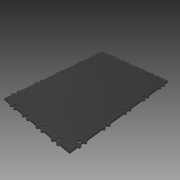
# Autodesk Inventor part: bottom
Saved by Autodesk Inventor 2014 (Build 180170000, 170)
## iProperties
Created: 2013-12-07
Part Number: bottom
Material: Generic
Document SubType Name: Modeling
Designer: buben
Density: 1 g/cm^3
Appearance: Anodized - Dark Gray
Author: buben
Subject: Laser Cutted
Autodesk Inventor part; units mm, degrees
ref_plane "YZ Plane" through (0, 0, 0) normal (1, 0, 0) x (0, 1, 0)
ref_plane "XZ Plane" through (0, 0, 0) normal (0, 1, 0) x (-1, 0, 0)
ref_plane "XY Plane" through (0, 0, 0) normal (0, 0, 1) x (1, 0, 0)
sketch "Sketch1" plane through (0, 0, 0) normal (0, 0, 1) x (1, 0, 0)
  line L0 (0, 0) -> (335, 0)
  line L1 (335, 0) -> (335, 489)
  line L2 (335, 489) -> (0, 489)
  line L3 (0, 489) -> (0, 0)
  dimension "d0" = 335
  dimension "d1" = 489
  constraints: 8 end point, 2 parallel, 1 horizontal, 1 perpendicular
  measures "d0" distance of L0.start L0.end
  measures "d1" distance of L2.end L0.start
extrude "Extrusion1" add sketch "Sketch1" along normal blind 6
sketch "Sketch6" plane through (0, 0, 6) normal (0, 0, 1) x (1, 0, 0)
  line L0 (0, 0) -> (335, 0) projected
  line L1 (335, 0) -> (335, 489) projected
  line L2 (335, 489) -> (0, 489) projected
  line L3 (0, 489) -> (0, 0) projected
  line L4 (55.45, 0) -> (59.95, 0)
  line L5 (59.95, 16.3) -> (55.45, 16.3)
  line L6 (62.45, 12.3) -> (62.45, 5)
  line L7 (52.95, 5) -> (52.95, 12.3)
  line L8 (55.45, 16.3) -> (55.45, 12.3)
  line L9 (55.45, 5) -> (55.45, 0)
  line L10 (59.95, 0) -> (59.95, 5)
  line L11 (59.95, 12.3) -> (59.95, 16.3)
  line L12 (62.45, 5) -> (59.95, 5)
  line L13 (55.45, 5) -> (52.95, 5)
  line L14 (52.95, 12.3) -> (55.45, 12.3)
  line L15 (59.95, 12.3) -> (62.45, 12.3)
  line L16 (128.65, 0) -> (133.15, 0)
  line L17 (133.15, 16.3) -> (128.65, 16.3)
  line L18 (135.65, 12.3) -> (135.65, 5)
  line L19 (126.15, 5) -> (126.15, 12.3)
  line L20 (128.65, 16.3) -> (128.65, 12.3)
  line L21 (128.65, 5) -> (128.65, 0)
  line L22 (133.15, 0) -> (133.15, 5)
  line L23 (133.15, 12.3) -> (133.15, 16.3)
  line L24 (135.65, 5) -> (133.15, 5)
  line L25 (128.65, 5) -> (126.15, 5)
  line L26 (126.15, 12.3) -> (128.65, 12.3)
  line L27 (133.15, 12.3) -> (135.65, 12.3)
  line L28 (201.85, 0) -> (206.35, 0)
  line L29 (206.35, 16.3) -> (201.85, 16.3)
  line L30 (208.85, 12.3) -> (208.85, 5)
  line L31 (199.35, 5) -> (199.35, 12.3)
  line L32 (201.85, 16.3) -> (201.85, 12.3)
  line L33 (201.85, 5) -> (201.85, 0)
  line L34 (206.35, 0) -> (206.35, 5)
  line L35 (206.35, 12.3) -> (206.35, 16.3)
  line L36 (208.85, 5) -> (206.35, 5)
  line L37 (201.85, 5) -> (199.35, 5)
  line L38 (199.35, 12.3) -> (201.85, 12.3)
  line L39 (206.35, 12.3) -> (208.85, 12.3)
  line L40 (275.05, 0) -> (279.55, 0)
  line L41 (279.55, 16.3) -> (275.05, 16.3)
  line L42 (282.05, 12.3) -> (282.05, 5)
  line L43 (272.55, 5) -> (272.55, 12.3)
  line L44 (275.05, 16.3) -> (275.05, 12.3)
  line L45 (275.05, 5) -> (275.05, 0)
  line L46 (279.55, 0) -> (279.55, 5)
  line L47 (279.55, 12.3) -> (279.55, 16.3)
  line L48 (282.05, 5) -> (279.55, 5)
  line L49 (275.05, 5) -> (272.55, 5)
  line L50 (272.55, 12.3) -> (275.05, 12.3)
  line L51 (279.55, 12.3) -> (282.05, 12.3)
  line L52 (0, 244.5) -> (335, 244.5) construction
  line L53 (55.45, 489) -> (59.95, 489)
  line L54 (59.95, 472.7) -> (55.45, 472.7)
  line L55 (62.45, 476.7) -> (62.45, 484)
  line L56 (52.95, 484) -> (52.95, 476.7)
  line L57 (55.45, 472.7) -> (55.45, 476.7)
  line L58 (55.45, 484) -> (55.45, 489)
  line L59 (59.95, 489) -> (59.95, 484)
  line L60 (59.95, 476.7) -> (59.95, 472.7)
  line L61 (62.45, 484) -> (59.95, 484)
  line L62 (55.45, 484) -> (52.95, 484)
  line L63 (52.95, 476.7) -> (55.45, 476.7)
  line L64 (59.95, 476.7) -> (62.45, 476.7)
  line L65 (128.65, 484) -> (126.15, 484)
  line L66 (135.65, 484) -> (133.15, 484)
  line L67 (128.65, 484) -> (128.65, 489)
  line L68 (128.65, 489) -> (133.15, 489)
  line L69 (133.15, 489) -> (133.15, 484)
  line L70 (126.15, 476.7) -> (128.65, 476.7)
  line L71 (126.15, 484) -> (126.15, 476.7)
  line L72 (133.15, 476.7) -> (135.65, 476.7)
  line L73 (135.65, 476.7) -> (135.65, 484)
  line L74 (128.65, 472.7) -> (128.65, 476.7)
  line L75 (133.15, 476.7) -> (133.15, 472.7)
  line L76 (133.15, 472.7) -> (128.65, 472.7)
  line L77 (201.85, 484) -> (199.35, 484)
  line L78 (208.85, 484) -> (206.35, 484)
  line L79 (201.85, 484) -> (201.85, 489)
  line L80 (201.85, 489) -> (206.35, 489)
  line L81 (206.35, 489) -> (206.35, 484)
  line L82 (199.35, 476.7) -> (201.85, 476.7)
  line L83 (199.35, 484) -> (199.35, 476.7)
  line L84 (206.35, 476.7) -> (208.85, 476.7)
  line L85 (208.85, 476.7) -> (208.85, 484)
  line L86 (201.85, 472.7) -> (201.85, 476.7)
  line L87 (206.35, 476.7) -> (206.35, 472.7)
  line L88 (206.35, 472.7) -> (201.85, 472.7)
  line L89 (275.05, 484) -> (272.55, 484)
  line L90 (282.05, 484) -> (279.55, 484)
  line L91 (275.05, 484) -> (275.05, 489)
  line L92 (275.05, 489) -> (279.55, 489)
  line L93 (279.55, 489) -> (279.55, 484)
  line L94 (272.55, 476.7) -> (275.05, 476.7)
  line L95 (272.55, 484) -> (272.55, 476.7)
  line L96 (279.55, 476.7) -> (282.05, 476.7)
  line L97 (282.05, 476.7) -> (282.05, 484)
  line L98 (275.05, 472.7) -> (275.05, 476.7)
  line L99 (279.55, 476.7) -> (279.55, 472.7)
  line L100 (279.55, 472.7) -> (275.05, 472.7)
  line L101 (16.3, 47.75) -> (16.3, 43.25)
  line L102 (0, 43.25) -> (0, 47.75)
  line L103 (5, 50.25) -> (12.3, 50.25)
  line L104 (12.3, 40.75) -> (5, 40.75)
  line L105 (5, 40.75) -> (5, 43.25)
  line L106 (5, 47.75) -> (5, 50.25)
  line L107 (12.3, 50.25) -> (12.3, 47.75)
  line L108 (12.3, 43.25) -> (12.3, 40.75)
  line L109 (0, 47.75) -> (5, 47.75)
  line L110 (12.3, 47.75) -> (16.3, 47.75)
  line L111 (16.3, 43.25) -> (12.3, 43.25)
  line L112 (5, 43.25) -> (0, 43.25)
  line L113 (167.5, 489) -> (167.5, 0) construction
  line L114 (16.3, 147.25) -> (16.3, 142.75)
  line L115 (0, 142.75) -> (0, 147.25)
  line L116 (5, 149.75) -> (12.3, 149.75)
  line L117 (12.3, 140.25) -> (5, 140.25)
  line L118 (5, 140.25) -> (5, 142.75)
  line L119 (5, 147.25) -> (5, 149.75)
  line L120 (12.3, 149.75) -> (12.3, 147.25)
  line L121 (12.3, 142.75) -> (12.3, 140.25)
  line L122 (0, 147.25) -> (5, 147.25)
  line L123 (12.3, 147.25) -> (16.3, 147.25)
  line L124 (16.3, 142.75) -> (12.3, 142.75)
  line L125 (5, 142.75) -> (0, 142.75)
  line L126 (16.3, 246.75) -> (16.3, 242.25)
  line L127 (0, 242.25) -> (0, 246.75)
  line L128 (5, 249.25) -> (12.3, 249.25)
  line L129 (12.3, 239.75) -> (5, 239.75)
  line L130 (5, 239.75) -> (5, 242.25)
  line L131 (5, 246.75) -> (5, 249.25)
  line L132 (12.3, 249.25) -> (12.3, 246.75)
  line L133 (12.3, 242.25) -> (12.3, 239.75)
  line L134 (0, 246.75) -> (5, 246.75)
  line L135 (12.3, 246.75) -> (16.3, 246.75)
  line L136 (16.3, 242.25) -> (12.3, 242.25)
  line L137 (5, 242.25) -> (0, 242.25)
  line L138 (16.3, 346.25) -> (16.3, 341.75)
  line L139 (0, 341.75) -> (0, 346.25)
  line L140 (5, 348.75) -> (12.3, 348.75)
  line L141 (12.3, 339.25) -> (5, 339.25)
  line L142 (5, 339.25) -> (5, 341.75)
  line L143 (5, 346.25) -> (5, 348.75)
  line L144 (12.3, 348.75) -> (12.3, 346.25)
  line L145 (12.3, 341.75) -> (12.3, 339.25)
  line L146 (0, 346.25) -> (5, 346.25)
  line L147 (12.3, 346.25) -> (16.3, 346.25)
  line L148 (16.3, 341.75) -> (12.3, 341.75)
  line L149 (5, 341.75) -> (0, 341.75)
  line L150 (16.3, 445.75) -> (16.3, 441.25)
  line L151 (0, 441.25) -> (0, 445.75)
  line L152 (5, 448.25) -> (12.3, 448.25)
  line L153 (12.3, 438.75) -> (5, 438.75)
  line L154 (5, 438.75) -> (5, 441.25)
  line L155 (5, 445.75) -> (5, 448.25)
  line L156 (12.3, 448.25) -> (12.3, 445.75)
  line L157 (12.3, 441.25) -> (12.3, 438.75)
  line L158 (0, 445.75) -> (5, 445.75)
  line L159 (12.3, 445.75) -> (16.3, 445.75)
  line L160 (16.3, 441.25) -> (12.3, 441.25)
  line L161 (5, 441.25) -> (0, 441.25)
  line L162 (318.7, 47.75) -> (318.7, 43.25)
  line L163 (335, 43.25) -> (335, 47.75)
  line L164 (330, 50.25) -> (322.7, 50.25)
  line L165 (322.7, 40.75) -> (330, 40.75)
  line L166 (330, 40.75) -> (330, 43.25)
  line L167 (330, 47.75) -> (330, 50.25)
  line L168 (322.7, 50.25) -> (322.7, 47.75)
  line L169 (322.7, 43.25) -> (322.7, 40.75)
  line L170 (335, 47.75) -> (330, 47.75)
  line L171 (322.7, 47.75) -> (318.7, 47.75)
  line L172 (318.7, 43.25) -> (322.7, 43.25)
  line L173 (330, 43.25) -> (335, 43.25)
  line L174 (322.7, 147.25) -> (318.7, 147.25)
  line L175 (318.7, 147.25) -> (318.7, 142.75)
  line L176 (318.7, 142.75) -> (322.7, 142.75)
  line L177 (322.7, 149.75) -> (322.7, 147.25)
  line L178 (322.7, 142.75) -> (322.7, 140.25)
  line L179 (322.7, 140.25) -> (330, 140.25)
  line L180 (330, 149.75) -> (322.7, 149.75)
  line L181 (330, 140.25) -> (330, 142.75)
  line L182 (330, 147.25) -> (330, 149.75)
  line L183 (335, 147.25) -> (330, 147.25)
  line L184 (335, 142.75) -> (335, 147.25)
  line L185 (330, 142.75) -> (335, 142.75)
  line L186 (322.7, 246.75) -> (318.7, 246.75)
  line L187 (318.7, 246.75) -> (318.7, 242.25)
  line L188 (318.7, 242.25) -> (322.7, 242.25)
  line L189 (322.7, 249.25) -> (322.7, 246.75)
  line L190 (322.7, 242.25) -> (322.7, 239.75)
  line L191 (322.7, 239.75) -> (330, 239.75)
  line L192 (330, 249.25) -> (322.7, 249.25)
  line L193 (330, 239.75) -> (330, 242.25)
  line L194 (330, 246.75) -> (330, 249.25)
  line L195 (335, 246.75) -> (330, 246.75)
  line L196 (335, 242.25) -> (335, 246.75)
  line L197 (330, 242.25) -> (335, 242.25)
  line L198 (322.7, 346.25) -> (318.7, 346.25)
  line L199 (318.7, 346.25) -> (318.7, 341.75)
  line L200 (318.7, 341.75) -> (322.7, 341.75)
  line L201 (322.7, 348.75) -> (322.7, 346.25)
  line L202 (322.7, 341.75) -> (322.7, 339.25)
  line L203 (322.7, 339.25) -> (330, 339.25)
  line L204 (330, 348.75) -> (322.7, 348.75)
  line L205 (330, 339.25) -> (330, 341.75)
  line L206 (330, 346.25) -> (330, 348.75)
  line L207 (335, 346.25) -> (330, 346.25)
  line L208 (335, 341.75) -> (335, 346.25)
  line L209 (330, 341.75) -> (335, 341.75)
  line L210 (322.7, 445.75) -> (318.7, 445.75)
  line L211 (318.7, 445.75) -> (318.7, 441.25)
  line L212 (318.7, 441.25) -> (322.7, 441.25)
  line L213 (322.7, 448.25) -> (322.7, 445.75)
  line L214 (322.7, 441.25) -> (322.7, 438.75)
  line L215 (322.7, 438.75) -> (330, 438.75)
  line L216 (330, 448.25) -> (322.7, 448.25)
  line L217 (330, 438.75) -> (330, 441.25)
  line L218 (330, 445.75) -> (330, 448.25)
  line L219 (335, 445.75) -> (330, 445.75)
  line L220 (335, 441.25) -> (335, 445.75)
  line L221 (330, 441.25) -> (335, 441.25)
  point P0 (57.7, 16.3)
  point P1 (130.9, 16.3)
  point P2 (204.1, 16.3)
  point P3 (277.3, 16.3)
  point P4 (57.7, 472.7)
  point P5 (130.9, 472.7)
  point P6 (204.1, 472.7)
  point P7 (277.3, 472.7)
  point P8 (16.3, 45.5)
  point P9 (16.3, 145)
  point P10 (16.3, 244.5)
  point P11 (16.3, 344)
  point P12 (16.3, 443.5)
  point P13 (318.7, 45.5)
  point P14 (318.7, 145)
  point P15 (318.7, 244.5)
  point P16 (318.7, 344)
  point P17 (318.7, 443.5)
  dimension "d66" = 4.5
  dimension "d67" = 7.3
  dimension "d68" = 5
  dimension "d69" = 4
  dimension "d70" = 2.5
  dimension "d71" = 2.5
  dimension "d72" = 57.7
  dimension "d75" = 73.2
  dimension "d80" = 4.5
  dimension "d81" = 7.3
  dimension "d82" = 5
  dimension "d83" = 4
  dimension "d84" = 2.5
  dimension "d85" = 2.5
  dimension "d86" = 45.5
  dimension "d89" = 99.5
  constraints: 436 end point, 117 symmetric about line, 20 parallel, 9 collinear, 8 perpendicular, 7 horizontal, 6 midpoint, 1 point on line, 1 vertical, 175 other
  measures "d66" distance of L5.start L5.end
  measures "d67" distance of L6.start L6.end
  measures "d68" distance of L4.end L10.end
  measures "d69" distance of L11.start L5.start
  measures "d70" distance of L7.end L8.end
  measures "d71" distance of L11.start L6.start
  measures "d72" distance from line of L3 point (57.7, 16.3)
  measures "d75" distance of L7.start L25.end
  measures "d80" distance of L101.start L101.end
  measures "d81" distance of L104.start L104.end
  measures "d82" distance of L105.end L102.start
  measures "d83" distance of L101.end L108.start
  measures "d84" distance of L104.end L105.end
  measures "d85" distance of L106.start L103.start
  measures "d86" distance from line of L0 point (16.3, 45.5)
  measures "d89" distance of L101.start L123.end
extrude "Extrusion6" cut sketch "Sketch6" against normal blind 6 contours L9 L13 L7 L14 L8 L5 L11 L15 L6 L12 L10 L0 | L3 L109 L106 L103 L107 L110 L101 L111 L108 L104 L105 L112 | L21 L25 L19 L26 L20 L17 L23 L27 L18 L24 L22 L0 | L3 L122 L119 L116 L120 L123 L114 L124 L121 L117 L118 L125 | L33 L37 L31 L38 L32 L29 L35 L39 L30 L36 L34 L0 | L3 L134 L131 L128 L132 L135 L126 L136 L133 L129 L130 L137 | L45 L49 L43 L50 L44 L41 L47 L51 L42 L48 L46 L0 | L3 L146 L143 L140 L144 L147 L138 L148 L145 L141 L142 L149 | L3 L158 L155 L152 L156 L159 L150 L160 L157 L153 L154 L161 | L173 L166 L165 L169 L172 L162 L171 L168 L164 L167 L170 L1 | L185 L181 L179 L178 L176 L175 L174 L177 L180 L182 L183 L1 | L2 L59 L61 L55 L64 L60 L54 L57 L63 L56 L62 L58 | L197 L193 L191 L190 L188 L187 L186 L189 L192 L194 L195 L1 | L2 L69 L66 L73 L72 L75 L76 L74 L70 L71 L65 L67 | L209 L205 L203 L202 L200 L199 L198 L201 L204 L206 L207 L1 | L2 L81 L78 L85 L84 L87 L88 L86 L82 L83 L77 L79 | L221 L217 L215 L214 L212 L211 L210 L213 L216 L218 L219 L1 | L2 L93 L90 L97 L96 L99 L100 L98 L94 L95 L89 L91
sketch "Sketch7" plane through (0, 0, 6) normal (0, 0, 1) x (1, 0, 0)
  line L0 (318.7, 242.25) -> (318.7, 246.75) projected
  line L1 (201.85, 489) -> (133.15, 489) projected
  line L2 (16.3, 246.75) -> (16.3, 242.25) projected
  line L3 (0, 142.75) -> (0, 47.75) projected
  line L4 (16.3, 47.75) -> (16.3, 43.25) projected
  line L5 (0, 43.25) -> (0, 0) projected
  line L6 (0, 0) -> (55.45, 0) projected
  line L7 (55.45, 16.3) -> (59.95, 16.3) projected
  line L8 (59.95, 0) -> (128.65, 0) projected
  line L9 (133.15, 0) -> (201.85, 0) projected
  line L10 (42.2, 0) -> (50.2, 0)
  line L11 (50.2, 0) -> (50.2, -4)
  line L12 (48.2, -6) -> (44.2, -6)
  line L13 (42.2, -4) -> (42.2, 0)
  line L14 (65.2, 0) -> (73.2, 0)
  line L15 (73.2, 0) -> (73.2, -4)
  line L16 (71.2, -6) -> (67.2, -6)
  line L17 (65.2, -4) -> (65.2, 0)
  line L18 (0, 38) -> (-4, 38)
  line L19 (-6, 36) -> (-6, 32)
  line L20 (-4, 30) -> (0, 30)
  line L21 (0, 30) -> (0, 38)
  line L22 (0, 61) -> (-4, 61)
  line L23 (-6, 59) -> (-6, 55)
  line L24 (-4, 53) -> (0, 53)
  line L25 (0, 53) -> (0, 61)
  arc A0 (-6, 55) -> (-4, 53) centre (-4, 55) ccw
  arc A1 (-4, 61) -> (-6, 59) centre (-4, 59) ccw
  arc A2 (-4, 38) -> (-6, 36) centre (-4, 36) ccw
  arc A3 (-6, 32) -> (-4, 30) centre (-4, 32) ccw
  arc A4 (42.2, -4) -> (44.2, -6) centre (44.2, -4) ccw
  arc A5 (48.2, -6) -> (50.2, -4) centre (48.2, -4) ccw
  arc A6 (65.2, -4) -> (67.2, -6) centre (67.2, -4) ccw
  arc A7 (71.2, -6) -> (73.2, -4) centre (71.2, -4) ccw
  line L26 (167.5, 489) -> (167.5, 0) construction
  line L27 (115.4, 0) -> (123.4, 0)
  line L28 (123.4, 0) -> (123.4, -4)
  line L29 (121.4, -6) -> (117.4, -6)
  line L30 (115.4, -4) -> (115.4, 0)
  line L31 (138.4, 0) -> (146.4, 0)
  line L32 (146.4, 0) -> (146.4, -4)
  line L33 (144.4, -6) -> (140.4, -6)
  line L34 (138.4, -4) -> (138.4, 0)
  arc A8 (115.4, -4) -> (117.4, -6) centre (117.4, -4) ccw
  arc A9 (121.4, -6) -> (123.4, -4) centre (121.4, -4) ccw
  arc A10 (138.4, -4) -> (140.4, -6) centre (140.4, -4) ccw
  arc A11 (144.4, -6) -> (146.4, -4) centre (144.4, -4) ccw
  line L35 (188.6, 0) -> (196.6, 0)
  line L36 (196.6, 0) -> (196.6, -4)
  line L37 (194.6, -6) -> (190.6, -6)
  line L38 (188.6, -4) -> (188.6, 0)
  line L39 (211.6, 0) -> (219.6, 0)
  line L40 (219.6, 0) -> (219.6, -4)
  line L41 (217.6, -6) -> (213.6, -6)
  line L42 (211.6, -4) -> (211.6, 0)
  arc A12 (188.6, -4) -> (190.6, -6) centre (190.6, -4) ccw
  arc A13 (194.6, -6) -> (196.6, -4) centre (194.6, -4) ccw
  arc A14 (211.6, -4) -> (213.6, -6) centre (213.6, -4) ccw
  arc A15 (217.6, -6) -> (219.6, -4) centre (217.6, -4) ccw
  line L43 (261.8, 0) -> (269.8, 0)
  line L44 (269.8, 0) -> (269.8, -4)
  line L45 (267.8, -6) -> (263.8, -6)
  line L46 (261.8, -4) -> (261.8, 0)
  line L47 (284.8, 0) -> (292.8, 0)
  line L48 (292.8, 0) -> (292.8, -4)
  line L49 (290.8, -6) -> (286.8, -6)
  line L50 (284.8, -4) -> (284.8, 0)
  arc A16 (261.8, -4) -> (263.8, -6) centre (263.8, -4) ccw
  arc A17 (267.8, -6) -> (269.8, -4) centre (267.8, -4) ccw
  arc A18 (284.8, -4) -> (286.8, -6) centre (286.8, -4) ccw
  arc A19 (290.8, -6) -> (292.8, -4) centre (290.8, -4) ccw
  line L51 (0, 137.5) -> (-4, 137.5)
  line L52 (-6, 135.5) -> (-6, 131.5)
  line L53 (-4, 129.5) -> (0, 129.5)
  line L54 (0, 129.5) -> (0, 137.5)
  line L55 (0, 160.5) -> (-4, 160.5)
  line L56 (-6, 158.5) -> (-6, 154.5)
  line L57 (-4, 152.5) -> (0, 152.5)
  line L58 (0, 152.5) -> (0, 160.5)
  arc A20 (-6, 154.5) -> (-4, 152.5) centre (-4, 154.5) ccw
  arc A21 (-4, 160.5) -> (-6, 158.5) centre (-4, 158.5) ccw
  arc A22 (-4, 137.5) -> (-6, 135.5) centre (-4, 135.5) ccw
  arc A23 (-6, 131.5) -> (-4, 129.5) centre (-4, 131.5) ccw
  line L59 (0, 237) -> (-4, 237)
  line L60 (-6, 235) -> (-6, 231)
  line L61 (-4, 229) -> (0, 229)
  line L62 (0, 229) -> (0, 237)
  line L63 (0, 260) -> (-4, 260)
  line L64 (-6, 258) -> (-6, 254)
  line L65 (-4, 252) -> (0, 252)
  line L66 (0, 252) -> (0, 260)
  arc A24 (-6, 254) -> (-4, 252) centre (-4, 254) ccw
  arc A25 (-4, 260) -> (-6, 258) centre (-4, 258) ccw
  arc A26 (-4, 237) -> (-6, 235) centre (-4, 235) ccw
  arc A27 (-6, 231) -> (-4, 229) centre (-4, 231) ccw
  line L67 (0, 336.5) -> (-4, 336.5)
  line L68 (-6, 334.5) -> (-6, 330.5)
  line L69 (-4, 328.5) -> (0, 328.5)
  line L70 (0, 328.5) -> (0, 336.5)
  line L71 (0, 359.5) -> (-4, 359.5)
  line L72 (-6, 357.5) -> (-6, 353.5)
  line L73 (-4, 351.5) -> (0, 351.5)
  line L74 (0, 351.5) -> (0, 359.5)
  arc A28 (-6, 353.5) -> (-4, 351.5) centre (-4, 353.5) ccw
  arc A29 (-4, 359.5) -> (-6, 357.5) centre (-4, 357.5) ccw
  arc A30 (-4, 336.5) -> (-6, 334.5) centre (-4, 334.5) ccw
  arc A31 (-6, 330.5) -> (-4, 328.5) centre (-4, 330.5) ccw
  line L75 (0, 436) -> (-4, 436)
  line L76 (-6, 434) -> (-6, 430)
  line L77 (-4, 428) -> (0, 428)
  line L78 (0, 428) -> (0, 436)
  line L79 (0, 459) -> (-4, 459)
  line L80 (-6, 457) -> (-6, 453)
  line L81 (-4, 451) -> (0, 451)
  line L82 (0, 451) -> (0, 459)
  arc A32 (-6, 453) -> (-4, 451) centre (-4, 453) ccw
  arc A33 (-4, 459) -> (-6, 457) centre (-4, 457) ccw
  arc A34 (-4, 436) -> (-6, 434) centre (-4, 434) ccw
  arc A35 (-6, 430) -> (-4, 428) centre (-4, 430) ccw
  line L83 (335, 38) -> (339, 38)
  line L84 (341, 36) -> (341, 32)
  line L85 (339, 30) -> (335, 30)
  line L86 (335, 30) -> (335, 38)
  line L87 (335, 61) -> (339, 61)
  line L88 (341, 59) -> (341, 55)
  line L89 (339, 53) -> (335, 53)
  line L90 (335, 53) -> (335, 61)
  arc A36 (339, 53) -> (341, 55) centre (339, 55) ccw
  arc A37 (341, 59) -> (339, 61) centre (339, 59) ccw
  arc A38 (341, 36) -> (339, 38) centre (339, 36) ccw
  arc A39 (339, 30) -> (341, 32) centre (339, 32) ccw
  line L91 (339, 152.5) -> (335, 152.5)
  line L92 (335, 160.5) -> (339, 160.5)
  line L93 (335, 152.5) -> (335, 160.5)
  arc A40 (341, 158.5) -> (339, 160.5) centre (339, 158.5) ccw
  line L94 (341, 158.5) -> (341, 154.5)
  arc A41 (339, 152.5) -> (341, 154.5) centre (339, 154.5) ccw
  arc A42 (341, 135.5) -> (339, 137.5) centre (339, 135.5) ccw
  line L95 (341, 135.5) -> (341, 131.5)
  arc A43 (339, 129.5) -> (341, 131.5) centre (339, 131.5) ccw
  line L96 (335, 137.5) -> (339, 137.5)
  line L97 (339, 129.5) -> (335, 129.5)
  line L98 (335, 129.5) -> (335, 137.5)
  line L99 (339, 252) -> (335, 252)
  line L100 (335, 260) -> (339, 260)
  line L101 (335, 252) -> (335, 260)
  arc A44 (341, 258) -> (339, 260) centre (339, 258) ccw
  line L102 (341, 258) -> (341, 254)
  arc A45 (339, 252) -> (341, 254) centre (339, 254) ccw
  arc A46 (341, 235) -> (339, 237) centre (339, 235) ccw
  line L103 (341, 235) -> (341, 231)
  arc A47 (339, 229) -> (341, 231) centre (339, 231) ccw
  line L104 (335, 237) -> (339, 237)
  line L105 (339, 229) -> (335, 229)
  line L106 (335, 229) -> (335, 237)
  line L107 (339, 351.5) -> (335, 351.5)
  line L108 (335, 359.5) -> (339, 359.5)
  line L109 (335, 351.5) -> (335, 359.5)
  arc A48 (341, 357.5) -> (339, 359.5) centre (339, 357.5) ccw
  line L110 (341, 357.5) -> (341, 353.5)
  arc A49 (339, 351.5) -> (341, 353.5) centre (339, 353.5) ccw
  arc A50 (341, 334.5) -> (339, 336.5) centre (339, 334.5) ccw
  line L111 (341, 334.5) -> (341, 330.5)
  arc A51 (339, 328.5) -> (341, 330.5) centre (339, 330.5) ccw
  line L112 (335, 336.5) -> (339, 336.5)
  line L113 (339, 328.5) -> (335, 328.5)
  line L114 (335, 328.5) -> (335, 336.5)
  line L115 (339, 451) -> (335, 451)
  line L116 (335, 459) -> (339, 459)
  line L117 (335, 451) -> (335, 459)
  arc A52 (341, 457) -> (339, 459) centre (339, 457) ccw
  line L118 (341, 457) -> (341, 453)
  arc A53 (339, 451) -> (341, 453) centre (339, 453) ccw
  arc A54 (341, 434) -> (339, 436) centre (339, 434) ccw
  line L119 (341, 434) -> (341, 430)
  arc A55 (339, 428) -> (341, 430) centre (339, 430) ccw
  line L120 (335, 436) -> (339, 436)
  line L121 (339, 428) -> (335, 428)
  line L122 (335, 428) -> (335, 436)
  line L123 (16.3, 244.5) -> (318.7, 244.5) construction
  line L124 (42.2, 489) -> (50.2, 489)
  line L125 (50.2, 489) -> (50.2, 493)
  line L126 (48.2, 495) -> (44.2, 495)
  line L127 (42.2, 493) -> (42.2, 489)
  line L128 (65.2, 489) -> (73.2, 489)
  line L129 (73.2, 489) -> (73.2, 493)
  line L130 (71.2, 495) -> (67.2, 495)
  line L131 (65.2, 493) -> (65.2, 489)
  arc A56 (44.2, 495) -> (42.2, 493) centre (44.2, 493) ccw
  arc A57 (50.2, 493) -> (48.2, 495) centre (48.2, 493) ccw
  arc A58 (67.2, 495) -> (65.2, 493) centre (67.2, 493) ccw
  arc A59 (73.2, 493) -> (71.2, 495) centre (71.2, 493) ccw
  line L132 (123.4, 489) -> (123.4, 493)
  arc A60 (123.4, 493) -> (121.4, 495) centre (121.4, 493) ccw
  line L133 (121.4, 495) -> (117.4, 495)
  arc A61 (117.4, 495) -> (115.4, 493) centre (117.4, 493) ccw
  line L134 (115.4, 489) -> (123.4, 489)
  line L135 (115.4, 493) -> (115.4, 489)
  line L136 (138.4, 493) -> (138.4, 489)
  arc A62 (140.4, 495) -> (138.4, 493) centre (140.4, 493) ccw
  line L137 (144.4, 495) -> (140.4, 495)
  line L138 (146.4, 489) -> (146.4, 493)
  arc A63 (146.4, 493) -> (144.4, 495) centre (144.4, 493) ccw
  line L139 (138.4, 489) -> (146.4, 489)
  line L140 (196.6, 489) -> (196.6, 493)
  arc A64 (196.6, 493) -> (194.6, 495) centre (194.6, 493) ccw
  line L141 (194.6, 495) -> (190.6, 495)
  arc A65 (190.6, 495) -> (188.6, 493) centre (190.6, 493) ccw
  line L142 (188.6, 489) -> (196.6, 489)
  line L143 (188.6, 493) -> (188.6, 489)
  line L144 (211.6, 493) -> (211.6, 489)
  arc A66 (213.6, 495) -> (211.6, 493) centre (213.6, 493) ccw
  line L145 (217.6, 495) -> (213.6, 495)
  line L146 (219.6, 489) -> (219.6, 493)
  arc A67 (219.6, 493) -> (217.6, 495) centre (217.6, 493) ccw
  line L147 (211.6, 489) -> (219.6, 489)
  line L148 (269.8, 489) -> (269.8, 493)
  arc A68 (269.8, 493) -> (267.8, 495) centre (267.8, 493) ccw
  line L149 (267.8, 495) -> (263.8, 495)
  arc A69 (263.8, 495) -> (261.8, 493) centre (263.8, 493) ccw
  line L150 (261.8, 489) -> (269.8, 489)
  line L151 (261.8, 493) -> (261.8, 489)
  line L152 (284.8, 493) -> (284.8, 489)
  arc A70 (286.8, 495) -> (284.8, 493) centre (286.8, 493) ccw
  line L153 (290.8, 495) -> (286.8, 495)
  line L154 (292.8, 489) -> (292.8, 493)
  arc A71 (292.8, 493) -> (290.8, 495) centre (290.8, 493) ccw
  line L155 (284.8, 489) -> (292.8, 489)
  point P0 (16.3, 45.5)
  point P1 (57.7, 16.3)
  dimension "d96" = 2
  dimension "d97" = 8
  dimension "d98" = 8
  dimension "d99" = 8
  dimension "d100" = 8
  dimension "d101" = 6
  dimension "d102" = 6
  dimension "d103" = 15
  dimension "d104" = 15
  dimension "d105" = 7.5
  dimension "d106" = 7.5
  dimension "d109" = 73.2
  dimension "d116" = 99.5
  constraints: 292 end point, 144 point on circle, 144 symmetric about line, 72 centre point, 16 tangent, 8 parallel, 7 equal radius, 6 midpoint, 5 horizontal, 4 perpendicular, 4 point on line, 2 collinear, 1 vertical, 232 other
  measures "d96" radius of A0
  measures "d97" distance between parallel lines of L24 L22
  measures "d98" distance between parallel lines of L20 L18
  measures "d99" distance between parallel lines of L11 L13
  measures "d100" distance between parallel lines of L15 L17
  measures "d101" distance between parallel lines of L3 L23
  measures "d102" distance between parallel lines of L6 L12
  measures "d103" distance between parallel lines of L18 L24
  measures "d104" distance between parallel lines of L17 L11
  measures "d105" distance from line of point (16.3, 45.5) L18
  measures "d106" distance from line of point (57.7, 16.3) L11
  measures "d109" distance of L10.end L28.start
  measures "d116" distance of L24.end L57.end
extrude "Extrusion7" add sketch "Sketch7" against normal blind 6
sketch "Sketch8" plane through (0, 0, 6) normal (0, 0, 1) x (1, 0, 0)
  line L0 (0, 129.5) -> (0, 61) projected
  line L1 (146.4, 0) -> (188.6, 0) projected
  circle A0 centre (176.5, 67.3) radius 2.25
  dimension "d123" = 4.5
  dimension "d124" = 67.3
  dimension "d125" = 176.5
  constraints: 1 centre point
  measures "d123" diameter of A0
  measures "d124" distance from line of L1 A0.centre
  measures "d125" distance from line of L0 A0.centre
extrude "Extrusion8" cut sketch "Sketch8" against normal through all
body "Solid1"
